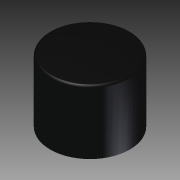
# Autodesk Inventor part: MBSCA
Saved by Autodesk Inventor 2015 (Build 190159000, 159)
## iProperties
Category: PARTsolutions
Company: NKKSWITCHES
Created: 2015-01-04
Part Number: MBSCA
Catalog Web Link: www.cadenas.de
Description: MB2000 Series - Bushing Mount Miniature Pushbuttons -caps-
Vendor: NKKSWITCHES
Document SubType Name: Modeling
Designer: PARTuser1
Manufacturer: NKKSWITCHES
Mass: 0.628922 g
Surface Area: 4.05412 cm^2
Volume: 0.628922 cm^3
Density: 1 g/cm^3
Material: Generic
Appearance: PSOLRGB-0-0-0
PSOL_IDENT_0: {$CADENAS_DATA\23d-libs\nkkswitches\pushbuttons\mb2000\parts\mb2000_bm_caps.prj},222 {VTYP=3D},{NB=M
PSOL_IDENT_1: BSCA},{LINA=MBSCA},{NN=MB2000 Series - Bushing Mount Miniature Pushbuttons -caps},{DATE=21.11.2014 0
PSOL_IDENT_2: 8:56:24},{GEOMDATE=15.12.2008 00:00:00},{VERSION=},{LINEID=10},{LINESUBID=-1},{WBVAR=PLNGRTYPS,CAPS,
PSOL_IDENT_3: CCLR}  {NB=MBSCA},{LINA=MBSCA},{KT=DUMMY},{PN=MBSCA},{SRS=MB},{PLNGRTYPS=S},{CAPS=C},{CCLR=A},{CCLRA
PSOL_IDENT_4: LG=0.00,0.00,0.00,0.00}
SUPPLIER: NKKSWITCHES
ARTICLENO: MBSCA
BOMINFO: MBSCA
CREATOR: CADENAS GmbH
Title: MBSCA
Author: Cadenas PARTsolutions
Autodesk Inventor part; units mm, degrees
sketch "Sketch_3" plane through (0, 0, 0) normal (1, 0, 0) x (0, 1, 0)
  line L0 (0, 0) -> (8.001, 0)
  line L1 (8.001, 0) -> (8.001, -4.7498)
  arc A0 (7.747, -5.0038) -> (8.001, -4.7498) centre (7.747, -4.7498) ccw
  line L2 (7.747, -5.0038) -> (0, -5.0038)
  line L3 (0, -5.0038) -> (0, 0)
  line L4 (0, 0) -> (8.001, 0)
  constraints: 10 end point, 2 point on circle, 1 centre point
revolve "Revolution1" add sketch "Sketch_3" angle 360 about axis through (0, 0, 0) along (0, -1, 0)
ref_plane "to_plunger_XY" through (0, 0, 0) normal (0, -1, 0) x (1, 0, 0)
ref_plane "to_plunger_YZ" through (0, 0, 0) normal (1, 0, 0) x (0, 0, 1)
ref_plane "to_plunger_ZX" through (0, 0, 0) normal (0, 0, 1) x (0, -1, 0)
body "Solid1"
